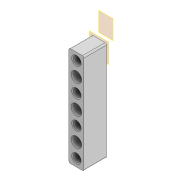
# Autodesk Inventor part: Omniscope_USBC_Bar_smallLenses
Saved by Autodesk Inventor 2022 (Build 260153000, 153)
## iProperties
Created: 2023-05-17
Part Number: Omniscope_USBC_Bar_smallLenses
Material: Generisch
Document SubType Name: Modeling
Designer: diederichbenedict
Density: 1 g/cm^3
Appearance: Vorgabe
Author: diederichbenedict
Autodesk Inventor part; units mm, degrees
ref_plane "YZ Plane" through (0, 0, 0) normal (1, 0, 0) x (0, 1, 0)
ref_plane "XZ Plane" through (0, 0, 0) normal (0, 1, 0) x (-1, 0, 0)
ref_plane "XY Plane" through (0, 0, 0) normal (0, 0, 1) x (1, 0, 0)
ref_plane "Arbeitsebene1" through (0, 0, 0) normal (0, 0, 1) x (1, 0, 0)
ref_plane "Arbeitsebene2" through (-1.5, 28.05, 3) normal (0, 0, 1) x (0, -1, 0)
sketch "Skizze2" plane through (-1.5, 28.05, 3) normal (0, 0, 1) x (0, -1, 0)
  circle A0 centre (56.1, 0) radius 4 construction
  circle A1 centre (56.1, 0) radius 4
  circle A2 centre (37.4, 0) radius 4 construction
  circle A3 centre (18.7, 0) radius 4 construction
  line L0 (6.2, -3) -> (-6.2, -3) construction
  circle A4 centre (0, 0) radius 4 construction
  circle A5 centre (37.4, 0) radius 4
  circle A6 centre (18.7, 0) radius 4
  circle A7 centre (0, 0) radius 4
  circle A8 centre (66, 1.5) radius 1.4 construction
  circle A9 centre (46.75, 1.5) radius 1.4 construction
  circle A10 centre (28.05, 1.5) radius 1.4 construction
  circle A11 centre (9.35, 1.5) radius 1.4 construction
  circle A12 centre (-9.9, 1.5) radius 1.4 construction
  circle A13 centre (66, 1.5) radius 1.6
  circle A14 centre (46.75, 1.5) radius 1.6
  circle A15 centre (28.05, 1.5) radius 1.6
  circle A16 centre (9.35, 1.5) radius 1.6
  circle A17 centre (-9.9, 1.5) radius 1.6
  line L1 (6, 6) -> (6, -6) projected
  line L2 (-6, 6) -> (6, 6) projected
  line L3 (-6, -6) -> (-6, 6) projected
  line L4 (6, -6) -> (-6, -6) projected
  circle A18 centre (0, 0) radius 4 projected
  line L5 (62.1, 6) -> (62.1, -6) projected
  line L6 (50.1, 6) -> (62.1, 6) projected
  line L7 (50.1, -6) -> (50.1, 6) projected
  line L8 (62.1, -6) -> (50.1, -6) projected
  circle A19 centre (56.1, 0) radius 4 projected
  line L9 (69.1, 6) -> (-12.4207, 6)
  line L10 (-12.4207, 6) -> (-12.4207, -6)
  line L11 (-12.4207, -6) -> (69.1, -6)
  line L12 (69.1, -6) -> (69.1, 6)
  circle A20 centre (66, 0) radius 1.6
  circle A21 centre (46.75, 0) radius 1.6
  circle A22 centre (28.05, 0) radius 1.6
  circle A23 centre (9.35, 0) radius 1.6031
  circle A24 centre (-9.9, 0) radius 1.6
  point P0 (28.05, 1.5)
  point P1 (50.1, 6)
  point P2 (6, 6)
  point P3 (6, -6)
  dimension "d0" = 8
  dimension "d1" = 8
  dimension "d2" = 8
  dimension "d3" = 8
  dimension "d4" = 3.2
  dimension "d5" = 3.2
  dimension "d6" = 3.2
  dimension "d7" = 3.2
  dimension "d8" = 3.2
  dimension "d9" = 7
  constraints: 14 centre point, 9 coincident, 8 end point, 2 parallel, 1 horizontal, 1 perpendicular, 2 other
  measures "d0" diameter of A1
  measures "d1" diameter of A5
  measures "d2" diameter of A6
  measures "d3" diameter of A7
  measures "d4" diameter of A13
  measures "d5" diameter of A14
  measures "d6" diameter of A15
  measures "d7" diameter of A16
  measures "d8" diameter of A17
  measures "d9" distance from line of L12 L5.start
extrude "Extrusion1" add sketch "Skizze2" along normal blind 10 contours A14 A21 | A15 A22 | A16 A23 | L9 L7 L11 L1 | L1 L4 L3 L2 | L6 L5 L8 L7 picked at (46.6839, 2.5883) picked at (27.9839, 2.5883) picked at (9.2849, 2.5894)
sketch "Skizze3" plane through (-1.5, 28.05, 13) normal (0, 0, 1) x (1, 0, 0)
  line L0 (-6, 6) -> (-6, -62.1) projected
  line L1 (-6, -62.1) -> (6, -62.1) projected
  line L2 (6, -62.1) -> (6, 6) projected
  line L3 (6, 6) -> (-6, 6) projected
  circle A0 centre (0, -18.7) radius 4 projected
  circle A1 centre (0, -37.4) radius 4 projected
  circle A2 centre (0, 0) radius 4 projected
  circle A3 centre (0, -56.1) radius 2.65
  circle A4 centre (0, -37.4) radius 4 projected
  circle A5 centre (0, -37.4) radius 2.65
  circle A6 centre (0, -18.7) radius 4 projected
  circle A7 centre (0, -18.7) radius 2.65
  circle A8 centre (0, 0) radius 2.65
  point P0 (1.5, -28.05)
  dimension "d12" = 5.3
  dimension "d13" = 5.3
  dimension "d14" = 5.3
  dimension "d15" = 5.3
  constraints: 4 centre point, 3 coincident
  measures "d12" diameter of A3
  measures "d13" diameter of A5
  measures "d14" diameter of A7
  measures "d15" diameter of A8
extrude "Extrusion2" add sketch "Skizze3" along normal blind 5 contours L3 L2 L1 L0 | A0 | A1 | A2
sketch "Skizze4" plane through (-1.5, 28.05, 18) normal (0, 0, 1) x (1, 0, 0)
  circle A0 centre (0, -46.75) radius 1.6 projected
  circle A1 centre (0, -28.05) radius 1.6 projected
  circle A2 centre (0, -9.35) radius 1.6031 projected
  point P0 (1.5, -28.05)
  point P1 (1.5, -46.75)
  point P2 (1.5, -28.05)
  point P3 (1.5, -9.35)
hole "Bohrung1" at (-1.5, -18.7, 18) at (-1.5, 0, 18) at (-1.5, 18.7, 18) direction (0, 0, -1) diameter 3.2 end through all counterbore diameter 7 counterbore depth 10
fillet "Rundung1" radius 2 4 edges at (4.5, -34.05, 10.5) (-7.5, -34.05, 10.5) (-7.5, 34.05, 10.5) (4.5, 34.05, 10.5)
chamfer "Fase1" distance 0.5 angle 45 4 edges at (-4.15, 28.05, 18) (-4.15, 9.35, 18) (-4.15, -9.35, 18) (-4.15, -28.05, 18)
chamfer "Fase2" distance 1.3 angle 45 3 edges at (-1.5, -5.35, 13) (-1.5, 13.35, 13) (-1.5, 32.05, 13)
sketch "Skizze5" plane through (-1.5, 28.05, 18) normal (0, 0, 1) x (1, 0, 0)
  circle A0 centre (0, -37.4) radius 3.15 projected
  circle A1 centre (0, 0) radius 3.15 projected
  circle A2 centre (0, -28.05) radius 3.5 projected
  circle A3 centre (0, -46.75) radius 3.5 projected
  circle A4 centre (0, -9.35) radius 3.5 projected
  arc A5 (6, 4) -> (4, 6) centre (4, 4) ccw projected
  line L0 (4, 6) -> (-4, 6) projected
  arc A6 (-4, 6) -> (-6, 4) centre (-4, 4) ccw projected
  line L1 (-6, 4) -> (-6, -60.1) projected
  arc A7 (-6, -60.1) -> (-4, -62.1) centre (-4, -60.1) ccw projected
  line L2 (-4, -62.1) -> (4, -62.1) projected
  arc A8 (4, -62.1) -> (6, -60.1) centre (4, -60.1) ccw projected
  line L3 (6, -60.1) -> (6, 4) projected
  circle A9 centre (0, -18.7) radius 3.15 projected
  circle A10 centre (0, -56.1) radius 3.15 projected
  line L4 (-5, -60.1) -> (-5, 4)
  arc A11 (-4, 5) -> (-5, 4) centre (-4, 4) ccw
  line L5 (-4, 5) -> (4, 5)
  arc A12 (5, 4) -> (4, 5) centre (4, 4) ccw
  line L6 (5, 4) -> (5, -60.1)
  arc A13 (4, -61.1) -> (5, -60.1) centre (4, -60.1) ccw
  line L7 (4, -61.1) -> (-4, -61.1)
  arc A14 (-5, -60.1) -> (-4, -61.1) centre (-4, -60.1) ccw
  point P0 (1.5, -28.05)
  dimension "d32" = 1
  constraints: 8 end point, 8 point on circle, 4 centre point, 7 other
  measures "d32" distance between parallel lines of L1 L4
extrude "Extrusion3" cut sketch "Skizze5" against normal through all contours L3 A8 L2 A7 L1 A6 L0 A5
equation "\"d0\" = d3"
equation "\"d1\" = d3"
equation "\"d2\" = d3"
equation "\"d12\" = d15"
equation "\"d13\" = d15"
equation "\"d14\" = d15"
